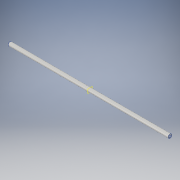
# Autodesk Inventor part: Churo_21_5_inches
Saved by Autodesk Inventor 2016 SP1 (Build 200210100, 210)
## iProperties
Created: 2016-02-04
Part Number: Churo_21_5_inches
Material: Aluminum 6061
Document SubType Name: Modeling
Designer: steele
Density: 2.7 g/cm^3
Appearance: Aluminum - Flat
Mass: 109.895 g
Surface Area: 244.736 cm^2
Volume: 40.702 cm^3
Author: steele
Autodesk Inventor part; units mm, degrees
ref_plane "XZ Plane" through (0, 0, 0) normal (0, 1, 0) x (-1, 0, 0)
ref_plane "XY Plane" through (0, 0, 0) normal (0, 0, 1) x (1, 0, 0)
sketch "Sketch1" plane through (0, 0, 0) normal (1, 0, 0) x (0, 1, 0)
  circle A0 centre (0, 0) radius 6.2865
  dimension "d1" = 12.573
  constraints: 1 centre point
  measures "d1" diameter of A0
extrude "Extrusion2" add sketch "Sketch1" along normal mid plane 546.1
sketch "Sketch2" plane through (-273.05, 0, 0) normal (-1, 0, 0) x (0, 0, 1)
  point P0 (0, 0)
  point P1 (0, 0)
  constraints: 1 coincident
hole "Hole1" at (-273.05, 0, 0) direction (1, 0, 0) diameter 5.8674 end through all
body "Solid2"
